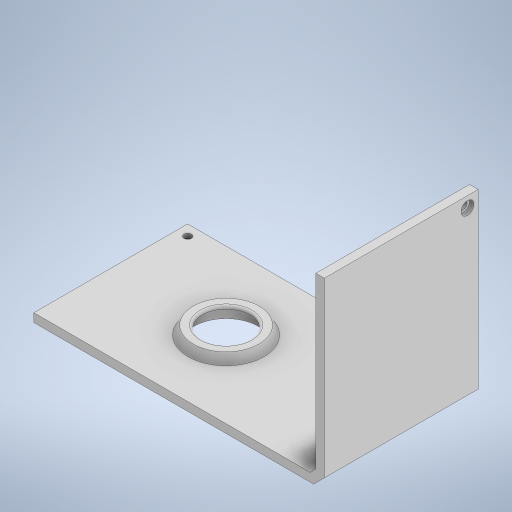
# Autodesk Inventor part: NOSS하단 커버
Saved by Autodesk Inventor 2023 (Build 270158000, 158)
## iProperties
Created: 2022-11-10
Part Number: NOSS하단 커버
Material: 일반
Document SubType Name: Modeling
Designer: user
Density: 1 g/cm^3
Appearance: 기본값
Author: user
Autodesk Inventor part; units mm, degrees
ref_plane "YZ Plane" through (0, 0, 0) normal (1, 0, 0) x (0, 1, 0)
ref_plane "XZ Plane" through (0, 0, 0) normal (0, 1, 0) x (-1, 0, 0)
ref_plane "XY Plane" through (0, 0, 0) normal (0, 0, 1) x (1, 0, 0)
sketch "스케치1" plane through (0, 0, 0) normal (0, 0, 1) x (1, 0, 0)
  line L0 (-70, 45) -> (70, 45)
  line L1 (70, 45) -> (70, -40)
  line L2 (65, -45) -> (-70, -45)
  line L3 (-70, -45) -> (-70, 45)
  line L4 (-70, 45) -> (70, -45) construction
  line L5 (70, 45) -> (-70, -45) construction
  line L6 (65, -45) -> (70, -40)
  line L7 (66, 41) -> (-66, 41)
  line L8 (-66, 41) -> (-66, -41)
  line L9 (-66, -41) -> (63.3431, -41)
  line L10 (63.3431, -41) -> (66, -38.3431)
  line L11 (66, -38.3431) -> (66, 41)
  line L12 (66, 41) -> (70, 41)
  line L13 (-66, -41) -> (-66, -45)
  point P0 (0, 0)
  dimension "d0" = 140
  dimension "d1" = 90
  dimension "d2" = 5
  dimension "d3" = 5
  dimension "d4" = 4
  constraints: 28 end point, 4 parallel, 4 point on line, 3 perpendicular, 2 horizontal, 2 midpoint, 4 other
  measures "d0" distance of L4.end L2.end
  measures "d1" distance of L0.end L4.end
  measures "d2" distance of L2.start L4.end
  measures "d3" distance of L1.end L4.end
  measures "d4" distance between parallel lines of L0 L7
extrude "돌출1" add sketch "스케치1" along normal blind 72 contours L1 L6 L2 L13 L9 L10 L11 L12
sketch "스케치2" plane through (66, -38.3431, 0) normal (-1, 0, 0) x (0, 0, 1)
  line L0 (15.5, 2.8431) -> (68.5, 2.8431) construction
  line L1 (68.5, 2.8431) -> (68.5, 71.8431) construction
  line L2 (68.5, 71.8431) -> (15.5, 71.8431) construction
  line L3 (15.5, 71.8431) -> (15.5, 2.8431) construction
  line L4 (15.5, 2.8431) -> (68.5, 71.8431) construction
  line L5 (68.5, 2.8431) -> (15.5, 71.8431) construction
  line L6 (68.5, -0.1569) -> (3.5, -0.1569)
  line L7 (3.5, -0.1569) -> (3.5, 79.8431)
  line L8 (3.5, 79.8431) -> (68.5, 79.8431)
  line L9 (68.5, 79.8431) -> (68.5, -0.1569) construction
  line L10 (68.5, -0.1569) -> (3.5, 79.8431) construction
  line L11 (3.5, -0.1569) -> (68.5, 79.8431) construction
  line L12 (72, 79.3431) -> (72, 0) projected
  line L13 (0, 79.3431) -> (72, 79.3431) projected
  circle A0 centre (35, 69.3431) radius 3
  circle A1 centre (61, 69.3431) radius 3
  circle A2 centre (18, 17.8431) radius 3
  circle A3 centre (66, 17.8431) radius 3
  point P0 (0, 38.3431)
  point P1 (42, 37.3431)
  point P2 (36, 39.8431)
  dimension "d7" = 53
  dimension "d8" = 69
  dimension "d9" = 80
  dimension "d10" = 65
  dimension "d11" = 3
  dimension "d12" = 30
  dimension "d13" = 42
  dimension "d14" = 6
  dimension "d15" = 6
  dimension "d16" = 6
  dimension "d17" = 6
  dimension "d18" = 2.5
  dimension "d19" = 2.5
  dimension "d21" = 26
  dimension "d22" = 15
  dimension "d23" = 15
  dimension "d24" = 2.5
  dimension "d25" = 2.5
  dimension "d35" = 7.5
  constraints: 24 end point, 4 centre point, 4 midpoint, 4 parallel, 2 horizontal, 2 perpendicular, 1 point on line
  measures "d7" distance of L2.end L1.end
  measures "d8" distance of L1.end L0.end
  measures "d9" distance of L8.end L6.start
  measures "d10" distance of L7.end L8.end
  measures "d11" distance between parallel lines of L6 L0
  measures "d12" distance from line of L12 point (42, 37.343)
  measures "d13" distance from line of L13 point (42, 37.343)
  measures "d14" diameter of A0
  measures "d15" diameter of A1
  measures "d16" diameter of A2
  measures "d17" diameter of A3
  measures "d18" distance from line of L2 A0.centre
  measures "d19" distance from line of L2 A1.centre
  measures "d21" distance of A1.centre A0.centre
  measures "d22" distance from line of L0 A2.centre
  measures "d23" distance from line of L0 A3.centre
  measures "d24" distance from line of L3 A2.centre
  measures "d25" distance from line of L1 A3.centre
  measures "d35" distance from line of L1 A1.centre
extrude "돌출2" add sketch "스케치2" along normal blind 3
sketch "스케치3" plane through (63, 31, 35) normal (-1, 0, 0) x (0, 0, 1)
  circle A0 centre (0, 0) radius 3 projected
  circle A1 centre (26, 0) radius 3 projected
  circle A2 centre (-17, -51.5) radius 3 projected
  circle A3 centre (31, -51.5) radius 3 projected
  point P0 (-35, -31)
hole "구멍1" at (63, 31, 35) at (63, -20.5, 18) at (63, -20.5, 66) at (63, 31, 61) direction (1, 0, 0) diameter 2 depth 5 tip angle 118 countersink diameter 3 countersink angle 90
ref_plane "작업 평면1" through (0, 0, 36) normal (0, 0, 1) x (1, 0, 0)
sketch "스케치5" plane through (0, 0, 36) normal (0, 0, 1) x (1, 0, 0)
  line L0 (-66, -45) -> (65, -45) projected
  line L1 (-12, -45) -> (-12, -15.6986)
  line L2 (70, -40) -> (70, 41) projected
  line L3 (-12, -45) -> (3, -45)
  line L4 (3, -45) -> (-1.6188, -37)
  line L5 (-1.6188, -37) -> (3.3812, -37)
  line L6 (3.3812, -37) -> (8, -45)
  line L7 (3, -45) -> (8, -45)
  line L8 (-1.6188, -37) -> (-12, -37)
  point P0 (0, 0)
  dimension "d37" = 82
  dimension "d38" = 5
  dimension "d39" = 40
  dimension "d40" = 60
  dimension "d41" = 8
  constraints: 14 end point, 4 point on line, 2 perpendicular, 1 collinear, 1 horizontal, 1 parallel
  measures "d37" distance between parallel lines of L2 L1
  measures "d38" distance of L4.end L5.end
  measures "d39" diameter of L6.end L1
  measures "d40" angle of L0 L4
  measures "d41" distance between parallel lines of L0 L5
revolve "회전1" add sketch "스케치5" angle 360 about axis through (-12, -45, 36) along (0, 1, 0) contours L4 L5 L6 L0
revolve "회전2" cut sketch "스케치5" angle 360 about axis through (-12, -45, 36) along (0, 1, 0) contours L1 L8 L4 L0
fillet "모깎기1" radius 1 1 edges at (-22.3812, -37, 36)
sketch "스케치6" plane through (-66, -41, 0) normal (0, 1, 0) x (1, 0, 0)
  line L0 (129, -25) -> (116, -25)
  line L1 (116, -25) -> (116, -38)
  line L2 (116, -38) -> (129, -38)
  line L3 (129, -38) -> (129, -25)
  line L4 (129, -25) -> (116, -38) construction
  line L5 (116, -25) -> (129, -38) construction
  line L6 (129, -63) -> (129, -69) projected
  line L7 (129, -66) -> (125.5723, -66)
  line L8 (129, -32) -> (129, -38) projected
  point P0 (66, 0)
  point P1 (122.5, -31.5)
  dimension "d45" = 28
  dimension "d46" = 13
  dimension "d47" = 13
  constraints: 14 end point, 3 midpoint, 2 horizontal, 2 parallel, 1 perpendicular, 1 point on line
  measures "d45" distance between parallel lines of L7 L2
  measures "d46" distance of L1.end L2.end
  measures "d47" distance of L0.end L1.end
extrude "돌출3" cut sketch "스케치6" against normal blind 19.25
sketch "스케치7" plane through (-66, -41, 0) normal (0, 1, 0) x (1, 0, 0)
  line L0 (126.5, -3) -> (118.5, -3)
  line L1 (118.5, -3) -> (118.5, -13)
  line L2 (118.5, -13) -> (126.5, -13)
  line L3 (126.5, -13) -> (126.5, -3)
  line L4 (126.5, -3) -> (118.5, -13) construction
  line L5 (118.5, -3) -> (126.5, -13) construction
  line L6 (116, -25) -> (129, -25) projected
  point P0 (66, 0)
  point P1 (122.5, -8)
  point P2 (122.5, -13)
  point P3 (122.5, -25)
  dimension "d51" = 8
  dimension "d52" = 10
  dimension "d53" = 12
  constraints: 12 end point, 4 midpoint, 2 parallel, 1 horizontal, 1 perpendicular, 1 vertical alignment
  measures "d51" distance of L2.end L1.end
  measures "d52" distance of L1.end L0.end
  measures "d53" distance between parallel lines of L6 L2
extrude "돌출4" cut sketch "스케치7" against normal blind 19.25
sketch "스케치8" plane through (-66, -41, 0) normal (0, 1, 0) x (1, 0, 0)
  circle A0 centre (111, -2.5) radius 2.5
  line L0 (113.5, 0) -> (108.5, 0)
  line L1 (108.5, 0) -> (108.5, -2.5)
  line L2 (108.5, -2.5) -> (113.5, -2.5)
  line L3 (113.5, -2.5) -> (113.5, 0)
  line L4 (113.5, 0) -> (108.5, -2.5) construction
  line L5 (108.5, 0) -> (113.5, -2.5) construction
  line L6 (129.3431, 0) -> (0, 0) projected
  line L7 (118.5, -13) -> (118.5, -3) projected
  point P0 (66, 0)
  point P1 (111, -1.25)
  point P2 (113.5, -2.5)
  dimension "d56" = 5
  dimension "d58" = 5
  constraints: 12 end point, 3 midpoint, 2 horizontal, 2 parallel, 1 coincident, 1 perpendicular, 1 point on line, 1 vertical alignment, 3 other
  measures "d58" distance between parallel lines of L7 L3
extrude "돌출5" cut sketch "스케치8" against normal blind 19.25
sketch "스케치9" plane through (-66, -45, 72) normal (0, -1, 0) x (1, 0, 0)
  circle A0 centre (5, -67) radius 1.75
  line L0 (0, -72) -> (108.5, -72) projected
  line L1 (0, -72) -> (0, 0) projected
  point P0 (66, -72)
  dimension "d61" = 3.5
  dimension "d62" = 5
  dimension "d63" = 5
  constraints: 1 centre point
  measures "d61" diameter of A0
  measures "d62" distance from line of L0 A0.centre
  measures "d63" distance from line of L1 A0.centre
extrude "돌출6" cut sketch "스케치9" against normal blind 19.25
sketch "스케치10" plane through (70, -40, 0) normal (1, 0, 0) x (0, 0, -1)
  circle A0 centre (-5, 76) radius 1.75
  line L0 (0, 0) -> (0, 81) projected
  line L1 (0, 81) -> (-72, 81) projected
  point P0 (0, 40)
  dimension "d66" = 3.5
  dimension "d67" = 5
  dimension "d68" = 5
  constraints: 1 centre point
  measures "d66" diameter of A0
  measures "d67" distance from line of L0 A0.centre
  measures "d68" distance from line of L1 A0.centre
extrude "돌출7" cut sketch "스케치10" against normal blind 19.25
sketch "스케치11" plane through (70, -40, 0) normal (1, 0, 0) x (0, 0, -1)
  circle A0 centre (-5, 76) radius 1.75 projected
  circle A1 centre (-5, 76) radius 3
  point P0 (0, 40)
  dimension "d71" = 6
  constraints: 1 centre point, 1 coincident
  measures "d71" diameter of A1
extrude "돌출8" cut sketch "스케치11" against normal blind 2 contours A0 | A1
sketch "스케치12" plane through (-66, -45, 72) normal (0, -1, 0) x (1, 0, 0)
  circle A0 centre (5, -67) radius 1.75 projected
  circle A1 centre (5, -67) radius 3
  point P0 (66, -72)
  dimension "d74" = 6
  constraints: 1 centre point, 1 coincident
  measures "d74" diameter of A1
extrude "돌출9" cut sketch "스케치12" against normal blind 2 contours A0 | A1
equation "\"d3\" = d2"
